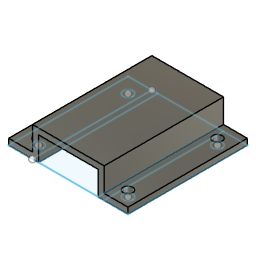
tunnel (Autodesk Fusion 360 design; units mm, degrees)
Autodesk Fusion 360 part; units mm, degrees
sketch "Sketch1" plane through (0, 0, 0) normal (0, 0, 1) x (1, 0, 0)
  line L0 (-100, 50) -> (-60, 50)
  line L1 (-60, 50) -> (-60, 10)
  line L2 (-60, 10) -> (-100, 10)
  line L3 (-100, 10) -> (-100, 50)
  line L4 (-90, 50) -> (-90, 10)
  line L5 (-70, 50) -> (-70, 10)
  circle A0 centre (-95, 15) radius 1.6
  circle A1 centre (-95, 45) radius 1.6
  circle A2 centre (-65, 45) radius 1.6
  circle A3 centre (-65, 15) radius 1.6
  line L6 (-68, 50) -> (-68, 10)
  line L7 (-92, 50) -> (-92, 10)
  dimension "d1" = 40
  dimension "d2" = 40
  dimension "d3" = 10
  dimension "d4" = 10
  dimension "d5" = 3.2
  dimension "d6" = 5
  dimension "d7" = 5
  dimension "d9" = 3.2
  dimension "d12" = 5
  dimension "d13" = 3.2
  dimension "d14" = 3.2
  dimension "d15" = 5
  dimension "d16" = 2
  constraint horizontal L0
  constraint vertical L1
  constraint horizontal L2
  constraint vertical L3
  constraint coincident L0 L4.start
  constraint coincident L2 L4.end
  constraint perpendicular L2 L4
  constraint coincident L0 L5.start
  constraint coincident L2 L5.end
  constraint perpendicular L2 L5
  constraint coincident L0 L6.start
  constraint coincident L2 L6.end
  constraint perpendicular L2 L6
  measures "d1" distance of L0.start L0.end
  measures "d2" distance of L0.end L1.end
  measures "d3" distance of L3 L4
  measures "d4" distance of L1 L5
  measures "d5" diameter of A0
  measures "d6" distance of L2 A0.centre
  measures "d7" distance of L3 A0.centre
  measures "d9" diameter of A1
  measures "d12" distance of L0 A1.centre
  measures "d13" diameter of A3
  measures "d14" diameter of A2
  measures "d15" distance of L1 A3.centre
  measures "d16" distance of L5 L6
extrude "Extrude1" add sketch "Sketch1" along normal blind 2 contours L0 L2 L3 L7 | L0 L1 L2 L6 makes body 1 at (-61.1861, 25.2314, 0) makes body 2 at (-98.8139, 34.7686, 0)
extrude "Extrude2" add sketch "Sketch1" along normal blind 12 contours L0 L2 L4 L7 | L0 L2 L5 L6 bodies 1 2
sketch "Sketch2" plane through (-90, 0, 0) normal (1, 0, 0) x (0, 1, 0)
  line L0 (10, 0) -> (50, 0)
  line L1 (50, 0) -> (50, 12)
  line L2 (50, 12) -> (10, 12)
  line L3 (10, 12) -> (10, 0)
  line L4 (10, 10) -> (50, 10)
  dimension "d21" = 2
  constraint coincident L3 L4.start
  constraint coincident L1 L4.end
  constraint perpendicular L1 L4
  measures "d21" distance of L2 L4
extrude "Extrude3" add sketch "Sketch2" along normal blind 20 contours L1 L2 L3 L4 bodies 1 2
extrude "Extrude4" add 1 faces at (-83.3333, 23.3333, 10) along direction (0, 0, -1) blind 2 on bodies 1 bodies 1
extrude "Extrude5" cut 1 faces at (-84, 36.6667, 12) along direction (0, 0, -1) blind 2 on bodies 1 bodies 1
